Autodesk Inventor part; units mm, degrees
(part 2 of 2)
sketch "Sketch7" plane through (0, 0, 3) normal (0, 0, 1) x (1, 0, 0)
  line L0 (156, -37.5) -> (158.9764, -37.8919) projected
  line L1 (156, -60.5) -> (156, -37.5)
  circle A0 centre (156, -49) radius 11.6
  point P0 (0, 0)
  dimension "d13" = 23.2
  constraints: 2 end point, 1 centre point, 1 midpoint, 1 vertical
  measures "d13" diameter of A0
extrude "Extrusion3" cut sketch "Sketch7" against normal through all
sketch "Sketch8" plane through (0, 0, 3) normal (0, 0, 1) x (1, 0, 0)
  point P0 (0, 0)
body "Solid1"
